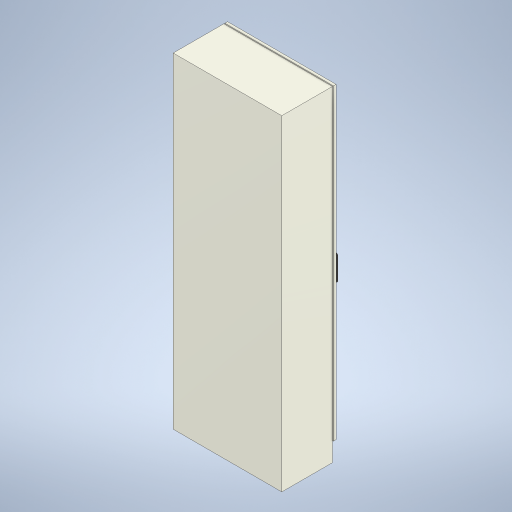
# Autodesk Inventor part: Schaltschrank2
Saved by Autodesk Inventor 2023 (Build 270158000, 158)
## iProperties
Created: 2025-06-27
Part Number: Schaltschrank2
Material: Generisch
Document SubType Name: Modeling
Designer: aurich
Density: 1 g/cm^3
Appearance: Vorgabe
Author: aurich
Autodesk Inventor part; units mm, degrees
ref_plane "YZ Plane" through (0, 0, 0) normal (1, 0, 0) x (0, 1, 0)
ref_plane "XZ Plane" through (0, 0, 0) normal (0, 1, 0) x (-1, 0, 0)
ref_plane "XY Plane" through (0, 0, 0) normal (0, 0, 1) x (1, 0, 0)
sketch "Skizze1" plane through (0, 0, 0) normal (0, 1, 0) x (-1, 0, 0)
  line L0 (0, 0) -> (600, 0)
  line L1 (600, 0) -> (600, -280)
  line L2 (600, -280) -> (0, -280)
  line L3 (0, -280) -> (0, 0)
  dimension "d0" = 600
  dimension "d1" = 280
  constraints: 8 end point, 2 parallel, 1 horizontal, 1 perpendicular
  measures "d0" distance of L1.end L2.end
  measures "d1" distance of L0.end L1.end
extrude "Extrusion1" add sketch "Skizze1" along normal blind 1800
sketch "Skizze2" plane through (0, 0, -280) normal (0, 0, -1) x (-1, 0, 0)
  line L0 (10, 1790) -> (590, 1790)
  line L1 (590, 1790) -> (590, 110)
  line L2 (590, 110) -> (10, 110)
  line L3 (10, 110) -> (10, 1790)
  line L4 (0, 0) -> (0, 1800) projected
  line L5 (600, 0) -> (600, 1800) projected
  line L6 (0, 1800) -> (600, 1800) projected
  line L7 (0, 0) -> (600, 0) projected
  dimension "d4" = 10
  dimension "d5" = 10
  dimension "d6" = 10
  dimension "d7" = 110
  constraints: 8 end point, 2 parallel, 1 horizontal, 1 perpendicular
  measures "d4" distance between parallel lines of L4 L3
  measures "d5" distance between parallel lines of L1 L5
  measures "d6" distance between parallel lines of L6 L0
  measures "d7" distance between parallel lines of L7 L2
extrude "Extrusion2" add sketch "Skizze2" along normal blind 5 contours L0 L1 L2 L3
sketch "Skizze3" plane through (0, 0, -285) normal (0, 0, -1) x (-1, 0, 0)
  line L0 (0, 0) -> (0, 1800) projected
  line L1 (600, 0) -> (600, 1800) projected
  line L2 (0, 1800) -> (600, 1800)
  line L3 (600, 1800) -> (600, 100)
  line L4 (600, 100) -> (0, 100)
  line L5 (0, 100) -> (0, 1800)
  line L6 (10, 110) -> (590, 110) projected
  point P0 (0, 100)
  dimension "d10" = 10
  constraints: 8 end point, 2 parallel, 1 horizontal, 1 perpendicular, 1 point on line
  measures "d10" distance between parallel lines of L4 L6
extrude "Extrusion3" add sketch "Skizze3" along normal blind 15
sketch "Skizze4" plane through (0, 0, -300) normal (0, 0, -1) x (-1, 0, 0)
  line L0 (15, 980) -> (25, 980)
  line L1 (35, 970) -> (35, 850)
  line L2 (25, 840) -> (15, 840)
  line L3 (5, 850) -> (5, 970)
  line L4 (0, 0) -> (600, 0) projected
  line L5 (0, 1800) -> (0, 100) projected
  arc A0 (5, 850) -> (15, 840) centre (15, 850) ccw
  arc A1 (25, 840) -> (35, 850) centre (25, 850) ccw
  arc A2 (35, 970) -> (25, 980) centre (25, 970) ccw
  arc A3 (15, 980) -> (5, 970) centre (15, 970) ccw
  dimension "d13" = 840
  dimension "d14" = 140
  dimension "d15" = 30
  dimension "d16" = 5
  dimension "d17" = 10
  constraints: 8 end point, 8 point on circle, 8 tangent, 4 centre point, 3 equal radius, 2 parallel, 1 horizontal, 1 perpendicular
  measures "d13" distance between parallel lines of L4 L2
  measures "d14" distance between parallel lines of L0 L2
  measures "d15" distance between parallel lines of L1 L3
  measures "d16" distance between parallel lines of L3 L5
  measures "d17" radius of A0
extrude "Extrusion4" add sketch "Skizze4" along normal blind 15
sketch "Skizze5" plane through (0, 0, -300) normal (0, 0, -1) x (-1, 0, 0)
  line L0 (150, 1140) -> (180, 1140)
  line L1 (180, 1140) -> (180, 1100)
  line L2 (180, 1100) -> (150, 1100)
  line L3 (150, 1100) -> (150, 1140)
  line L4 (0, 100) -> (600, 100) projected
  line L5 (0, 1800) -> (0, 100) projected
  line L6 (240, 1140) -> (270, 1140)
  line L7 (270, 1140) -> (270, 1100)
  line L8 (270, 1100) -> (240, 1100)
  line L9 (240, 1100) -> (240, 1140)
  line L10 (330, 1140) -> (360, 1140)
  line L11 (360, 1140) -> (360, 1100)
  line L12 (360, 1100) -> (330, 1100)
  line L13 (330, 1100) -> (330, 1140)
  line L14 (420, 1140) -> (450, 1140)
  line L15 (450, 1140) -> (450, 1100)
  line L16 (450, 1100) -> (420, 1100)
  line L17 (420, 1100) -> (420, 1140)
  line L18 (150, 1050) -> (180, 1050)
  line L19 (180, 1050) -> (180, 1010)
  line L20 (180, 1010) -> (150, 1010)
  line L21 (150, 1010) -> (150, 1050)
  line L22 (240, 1050) -> (270, 1050)
  line L23 (270, 1050) -> (270, 1010)
  line L24 (270, 1010) -> (240, 1010)
  line L25 (240, 1010) -> (240, 1050)
  line L26 (330, 1050) -> (360, 1050)
  line L27 (360, 1050) -> (360, 1010)
  line L28 (360, 1010) -> (330, 1010)
  line L29 (330, 1010) -> (330, 1050)
  line L30 (420, 1050) -> (450, 1050)
  line L31 (450, 1050) -> (450, 1010)
  line L32 (450, 1010) -> (420, 1010)
  line L33 (420, 1010) -> (420, 1050)
  line L34 (250, 960) -> (350, 960)
  line L35 (350, 960) -> (350, 860)
  line L36 (350, 860) -> (250, 860)
  line L37 (250, 860) -> (250, 960)
  point P0 (0, 0)
  dimension "d20" = 40
  dimension "d21" = 30
  dimension "d22" = 1000
  dimension "d23" = 150
  dimension "d33" = 90
  dimension "d36" = 90
  dimension "d39" = 100
  dimension "d40" = 100
  dimension "d41" = 250
  dimension "d42" = 50
  constraints: 72 end point, 4 parallel, 3 horizontal, 2 collinear, 2 perpendicular, 1 vertical, 54 other
  measures "d20" distance between parallel lines of L2 L0
  measures "d21" distance between parallel lines of L1 L3
  measures "d22" distance between parallel lines of L4 L2
  measures "d23" distance between parallel lines of L5 L3
  measures "d33" distance of L0.start L6.start
  measures "d36" distance of L0.start L18.start
  measures "d39" distance of L35.end L36.end
  measures "d40" distance of L34.end L35.end
  measures "d41" distance between parallel lines of L5 L37
  measures "d42" distance between parallel lines of L20 L34
extrude "Extrusion5" add sketch "Skizze5" along normal blind 5
sketch "Skizze6" plane through (0, 0, -305) normal (0, 0, -1) x (-1, 0, 0)
  circle A0 centre (165, 1120) radius 12.5
  line L0 (180, 1140) -> (150, 1140) projected
  line L1 (180, 1100) -> (180, 1140) projected
  circle A1 centre (255, 1120) radius 12.5
  circle A2 centre (345, 1120) radius 12.5
  circle A3 centre (435, 1120) radius 12.5
  circle A4 centre (165, 1030) radius 12.5
  circle A5 centre (255, 1030) radius 12.5
  circle A6 centre (345, 1030) radius 12.5
  circle A7 centre (435, 1030) radius 12.5
  circle A8 centre (300, 910) radius 50
  line L2 (350, 860) -> (350, 960) projected
  line L3 (350, 960) -> (250, 960) projected
  arc A9 (308, 866.7334) -> (292, 866.7334) centre (300, 910) ccw
  line L4 (292, 915) -> (292, 866.7334)
  line L5 (308, 915) -> (308, 866.7334)
  line L6 (292, 915) -> (300, 923)
  line L7 (292, 915) -> (303.3137, 915) construction
  line L8 (308, 915) -> (300, 923)
  line L9 (308, 915) -> (319.3137, 915) construction
  point P0 (0, 0)
  dimension "d45" = 25
  dimension "d46" = 20
  dimension "d47" = 15
  dimension "d50" = 90
  dimension "d53" = 90
  dimension "d68" = 100
  dimension "d69" = 88
  dimension "d70" = 45
  dimension "d71" = 135
  dimension "d72" = 8
  dimension "d73" = 8
  dimension "d74" = 5
  constraints: 12 end point, 10 centre point, 3 horizontal, 3 vertical, 2 equal length, 2 point on circle, 2 tangent, 1 coincident, 1 horizontal alignment, 14 other
  measures "d45" diameter of A0
  measures "d46" distance from line of L0 A0.centre
  measures "d47" distance from line of L1 A0.centre
  measures "d50" distance of A0.centre A1.centre
  measures "d53" distance of A0.centre A4.centre
  measures "d68" diameter of A8
  measures "d69" diameter of A9
  measures "d70" angle of L7 L6
  measures "d71" angle of L9 L8
  measures "d72" distance from line of L5 A8.centre
  measures "d73" distance from line of A8.centre L4
  measures "d74" vertical distance of A8.centre L5.start
extrude "Extrusion6" add sketch "Skizze6" along normal blind 10 contours A0 | A1 | A2 | A3 | A4 | A5 | A6 | A7 | A8
sketch "Skizze7" plane through (0, 0, -305) normal (0, 0, -1) x (-1, 0, 0)
  line L0 (292, 942) -> (308, 942)
  line L1 (308, 942) -> (308, 930)
  line L2 (308, 930) -> (292, 930)
  line L3 (292, 930) -> (292, 942)
  line L4 (308, 866.7334) -> (308, 915) projected
  line L5 (292, 915) -> (292, 866.7334) projected
  point P0 (0, 0)
  point P1 (300, 923)
  dimension "d75" = 7
  dimension "d76" = 12
  constraints: 8 end point, 2 parallel, 2 point on line, 1 horizontal, 1 perpendicular
  measures "d75" distance from line of point (300, 923) L2
  measures "d76" distance between parallel lines of L2 L0
extrude "Extrusion7" cut sketch "Skizze7" against normal blind 1
equation "\"d5\" = d4"
equation "\"d6\" = d5"
equation "\"d73\" = d72"
